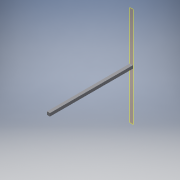
# Autodesk Inventor part: Ross Rail
Saved by Autodesk Inventor 2016 (Build 200138000, 138)
## iProperties
Created: 2016-05-31
Part Number: Ross Rail
Material: Generic
Document SubType Name: Modeling
Designer: Scott
Density: 1 g/cm^3
Appearance: Default
Author: Scott
Autodesk Inventor part; units mm, degrees
ref_plane "YZ Plane" through (0, 0, 0) normal (1, 0, 0) x (0, 1, 0)
ref_plane "XZ Plane" through (0, 0, 0) normal (0, 1, 0) x (-1, 0, 0)
ref_plane "Work Plane1" through (0, 0, 0) normal (0, 0, 1) x (1, 0, 0)
sketch "Sketch1" plane through (0, 0, 0) normal (0, 0, 1) x (1, 0, 0)
  line L0 (-3.175, 609.6) -> (-3.175, 0) projected
  line L1 (-3.175, 609.6) -> (-23.175, 609.6) projected
  line L2 (-23.175, 0) -> (-23.175, 609.6) projected
  line L3 (-3.175, 0) -> (-23.175, 0) projected
  line L4 (-3.175, 314.8) -> (-23.175, 314.8)
  line L5 (-23.175, 314.8) -> (-23.175, 294.8)
  line L6 (-23.175, 294.8) -> (-3.175, 294.8)
  line L7 (-3.175, 294.8) -> (-3.175, 314.8)
  line L8 (-3.175, 314.8) -> (-23.175, 294.8) construction
  line L9 (-23.175, 314.8) -> (-3.175, 294.8) construction
  point P0 (0, 0)
  point P1 (-13.175, 304.8)
  dimension "d0" = 20
  dimension "d1" = 20
  constraints: 12 end point, 2 midpoint, 2 parallel, 1 horizontal, 1 perpendicular
  measures "d0" distance of L6.end L5.end
  measures "d1" distance of L5.end L4.end
ref_plane "Work Plane2" through (-23.175, 0, 558.8) normal (0, 0, -1) x (0, 1, 0)
extrude "Extrusion1" add sketch "Sketch1" along normal up to surface (558.8 mm away) contours L0 L6 L2 L4
body "Solid1"
